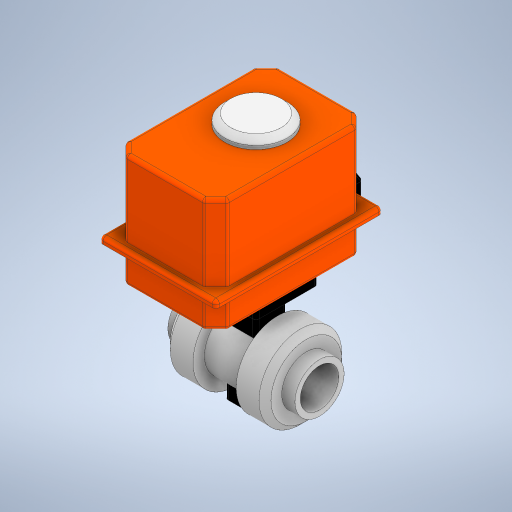
# Autodesk Inventor part: СДР 080 Электроклапан
Saved by Autodesk Inventor 2024.2 (Build 282272000, 272)
## iProperties
Created: 2024-04-05
Part Number: СДР 080 Электроклапан
Material: Generic
Document SubType Name: Modeling
Designer: pokla
Density: 1 g/cm^3
Appearance: Default
Author: pokla
Autodesk Inventor part; units mm, degrees
ref_plane "YZ Plane" through (0, 0, 0) normal (1, 0, 0) x (0, 1, 0)
ref_plane "XZ Plane" through (0, 0, 0) normal (0, 1, 0) x (-1, 0, 0)
ref_plane "XY Plane" through (0, 0, 0) normal (0, 0, 1) x (1, 0, 0)
sketch "Sketch1" plane through (0, 0, 0) normal (0, 1, 0) x (-1, 0, 0)
  line L0 (1079.5, -1295.4) -> (-1079.5, -1295.4)
  line L1 (-1079.5, -1295.4) -> (-1079.5, 1930.4)
  line L2 (-1079.5, 1930.4) -> (1079.5, 1930.4)
  line L3 (1079.5, 1930.4) -> (1079.5, -1295.4)
  line L4 (-1231.9, -1447.8) -> (1231.9, -1447.8)
  line L5 (1231.9, -1447.8) -> (1231.9, 2082.8)
  line L6 (1231.9, 2082.8) -> (-1231.9, 2082.8)
  line L7 (-1231.9, 2082.8) -> (-1231.9, -1447.8)
  point P0 (0, 0)
  point P1 (0, -1295.4)
  dimension "d0" = 2159
  dimension "d1" = 3225.8
  dimension "d5" = 1295.4
  dimension "d6" = 152.4
  constraints: 16 end point, 4 parallel, 2 perpendicular, 1 horizontal, 1 midpoint, 1 vertical alignment, 3 other
  measures "d0" distance of L1.end L2.end
  measures "d1" distance of L0.end L1.end
  measures "d5" distance of point (0, 0) point (0, -1295.4)
  measures "d6" distance between parallel lines of L0 L4
extrude "Extrusion1" add sketch "Sketch1" along normal mid plane 139.7 contours L0 L1 L2 L3 | L7 L6 L5 L4
sketch "Sketch2" plane through (0, 0, 0) normal (0, 1, 0) x (-1, 0, 0)
  line L0 (1231.9, -1447.8) -> (1231.9, 2082.8) projected
  line L1 (1231.9, 2082.8) -> (-1231.9, 2082.8) projected
  line L2 (-1231.9, 2082.8) -> (-1231.9, -1447.8) projected
  line L3 (-1231.9, -1447.8) -> (1231.9, -1447.8) projected
  line L4 (1079.5, -1295.4) -> (1079.5, 1930.4)
  line L5 (1079.5, 1930.4) -> (-1079.5, 1930.4)
  line L6 (-1079.5, 1930.4) -> (-1079.5, -1295.4)
  line L7 (-1079.5, -1295.4) -> (1079.5, -1295.4)
  point P0 (0, 0)
  dimension "d9" = 152.4
  constraints: 8 end point, 3 other
  measures "d9" distance between parallel lines of L3 L7
extrude "Extrusion2" add sketch "Sketch2" along normal blind 1676.4 and the other way blind 736.6 contours L7 L6 L5 L4
sketch "Sketch3" plane through (0, 0, 0) normal (0, 1, 0) x (-1, 0, 0)
  circle A0 centre (0, 0) radius 660.4
  line L0 (1231.9, -1447.8) -> (-1231.9, -1447.8) projected
  line L1 (1079.5, 1930.4) -> (-1079.5, 1930.4) projected
  line L2 (-1079.5, 1930.4) -> (-1079.5, -1295.4) projected
  line L3 (-1079.5, -1295.4) -> (1079.5, -1295.4) projected
  line L4 (1079.5, -1295.4) -> (1079.5, 1930.4) projected
  point P0 (0, 0)
  point P1 (0, -1447.8)
  point P2 (0, -1295.4)
  dimension "d14" = 1320.8
  dimension "d16" = 1295.4
  constraints: 2 midpoint, 1 centre point, 1 coincident
  measures "d14" diameter of A0
  measures "d16" distance of A0.centre point (0, -1295.4)
extrude "Extrusion3" add sketch "Sketch3" along normal blind 1879.6 and the other way blind 12.7 contours A0
sketch "Sketch4" plane through (0, 0, 0) normal (0, 1, 0) x (-1, 0, 0)
  line L0 (685.8, -685.8) -> (-685.8, -685.8)
  line L1 (-685.8, -685.8) -> (-685.8, 685.8)
  line L2 (-685.8, 685.8) -> (685.8, 685.8)
  line L3 (685.8, 685.8) -> (685.8, -685.8)
  circle A0 centre (0, 0) radius 660.4 projected
  line L4 (1079.5, 1930.4) -> (-1079.5, 1930.4) projected
  line L5 (-1079.5, 1930.4) -> (-1079.5, -1295.4) projected
  line L6 (-1079.5, -1295.4) -> (1079.5, -1295.4) projected
  line L7 (1079.5, -1295.4) -> (1079.5, 1930.4) projected
  point P0 (0, 0)
  point P1 (0, -685.8)
  point P2 (0, -1295.4)
  dimension "d21" = 1371.6
  dimension "d22" = 1371.6
  dimension "d23" = 609.6
  constraints: 8 end point, 2 midpoint, 2 parallel, 1 horizontal, 1 perpendicular, 1 vertical alignment
  measures "d21" distance of L1.end L2.end
  measures "d22" distance of L0.end L1.end
  measures "d23" distance of point (0, -685.8) point (0, -1295.4)
extrude "Extrusion4" add sketch "Sketch4" against normal blind 990.6 contours L0 L1 L2 L3 | A0
sketch "Sketch5" plane through (0, 0, 0) normal (0, 1, 0) x (-1, 0, 0)
  line L0 (-685.8, 685.8) -> (685.8, 685.8) projected
  line L1 (685.8, 685.8) -> (685.8, -685.8) projected
  line L2 (685.8, -685.8) -> (-685.8, -685.8) projected
  line L3 (-685.8, -685.8) -> (-685.8, 685.8) projected
  line L4 (-660.4, -660.4) -> (660.4, -660.4)
  line L5 (660.4, -660.4) -> (660.4, 660.4)
  line L6 (660.4, 660.4) -> (-660.4, 660.4)
  line L7 (-660.4, 660.4) -> (-660.4, -660.4)
  point P0 (0, 0)
  dimension "d26" = 25.4
  constraints: 8 end point, 3 other
  measures "d26" distance between parallel lines of L2 L4
extrude "Extrusion5" add sketch "Sketch5" against normal blind 1270 contours L7 L6 L5 L4
sketch "Sketch6" plane through (0, 0, 0) normal (0, 1, 0) x (-1, 0, 0)
  line L0 (660.4, 660.4) -> (660.4, -660.4) projected
  line L1 (660.4, -660.4) -> (-660.4, -660.4) projected
  line L2 (-660.4, -660.4) -> (-660.4, 660.4) projected
  line L3 (-660.4, 660.4) -> (660.4, 660.4) projected
  line L4 (-330.2, -330.2) -> (330.2, -330.2)
  line L5 (330.2, -330.2) -> (330.2, 330.2)
  line L6 (330.2, 330.2) -> (-330.2, 330.2)
  line L7 (-330.2, 330.2) -> (-330.2, -330.2)
  point P0 (0, 0)
  dimension "d29" = 330.2
  constraints: 8 end point, 3 other
  measures "d29" distance between parallel lines of L1 L4
extrude "Extrusion6" add sketch "Sketch6" against normal blind 3352.8 contours L7 L6 L5 L4
sketch "Sketch7" plane through (0, 0, 0) normal (1, 0, 0) x (0, 1, 0)
  line L0 (-1270, -330.2) -> (-1270, 330.2) projected
  line L1 (-1270, -330.2) -> (-3352.8, -330.2) projected
  line L2 (-3352.8, 330.2) -> (-3352.8, -330.2) projected
  line L3 (-1270, 330.2) -> (-3352.8, 330.2) projected
  circle A0 centre (-2489.2, 0) radius 635
  point P0 (0, 0)
  point P1 (-1270, 0)
  dimension "d32" = 1270
  dimension "d33" = 1219.2
  constraints: 1 centre point, 1 horizontal alignment, 1 midpoint
  measures "d32" diameter of A0
  measures "d33" distance of point (-1270, 0) A0.centre
extrude "Extrusion7" add sketch "Sketch7" along normal mid plane 914.4 contours A0 L1 | L1 A0 L3 | L3 A0
sketch "Sketch8" plane through (0, 0, 0) normal (1, 0, 0) x (0, 1, 0)
  circle A0 centre (-2489.2, 0) radius 635 projected
  circle A1 centre (-2489.2, 0) radius 406.4
  circle A2 centre (-2489.2, 0) radius 520.7
  point P0 (0, 0)
  dimension "d36" = 812.8
  dimension "d37" = 1041.4
  constraints: 2 centre point, 2 coincident
  measures "d36" diameter of A1
  measures "d37" diameter of A2
extrude "Extrusion8" add sketch "Sketch8" along normal mid plane 2692.4 contours A2
sketch "Sketch9" plane through (-457.2, -2489.2, 0) normal (-1, 0, 0) x (0, 0, 1)
  circle A0 centre (0, 0) radius 406.4 projected
  circle A1 centre (0, 0) radius 876.3
  point P0 (0, 2489.2)
  dimension "d40" = 1752.6
  constraints: 1 centre point, 1 coincident
  measures "d40" diameter of A1
extrude "Extrusion9" add sketch "Sketch9" along normal blind 609.6
chamfer "Chamfer1" distance 127 angle 45 1 edges at (-1066.8, -2489.2, -876.3)
mirror "Mirror1" about plane through (0, 0, 0) normal (1, 0, 0) of "Extrusion9", "Chamfer1"
sketch "Sketch10" plane through (0, 0, 0) normal (0, 0, 1) x (1, 0, 0)
  line L0 (-1231.9, -69.85) -> (1231.9, -69.85) projected
  line L1 (1079.5, -69.85) -> (-1079.5, -69.85) projected
  line L2 (1079.5, -736.6) -> (1079.5, -69.85) projected
  line L3 (-1079.5, -736.6) -> (1079.5, -736.6) projected
  line L4 (-1079.5, -736.6) -> (-1079.5, -69.85) projected
  line L5 (304.8, -69.85) -> (304.8, -374.65)
  arc A0 (-304.8, -374.65) -> (304.8, -374.65) centre (0, -374.65) ccw
  line L6 (-304.8, -374.65) -> (-304.8, -69.85)
  point P0 (0, 0)
  point P1 (0, -679.45)
  point P2 (0, -69.85)
  point P3 (-304.8, -69.85)
  dimension "d46" = 609.6
  dimension "d47" = 609.6
  constraints: 4 end point, 3 point on circle, 2 perpendicular, 2 point on line, 2 tangent, 1 centre point, 1 midpoint, 1 vertical alignment
  measures "d46" distance between parallel lines of L6 L5
  measures "d47" distance of point (0, -69.85) point (0, -679.45)
extrude "Extrusion10" add sketch "Sketch10" against normal blind 1422.4 contours L0 L5 A0 L6
sketch "Sketch11" plane through (0, 0, 0) normal (0, 0, 1) x (1, 0, 0)
  line L0 (304.8, -69.85) -> (304.8, -374.65) projected
  arc A0 (-304.8, -374.65) -> (304.8, -374.65) centre (0, -374.65) ccw projected
  line L1 (-304.8, -374.65) -> (-304.8, -69.85) projected
  line L2 (304.8, -69.85) -> (-304.8, -69.85) projected
  line L3 (0, -66.6914) -> (266.7, -220.6707)
  line L4 (266.7, -220.6707) -> (266.7, -528.6293)
  line L5 (266.7, -528.6293) -> (0, -682.6086)
  line L6 (0, -682.6086) -> (-266.7, -528.6293)
  line L7 (-266.7, -528.6293) -> (-266.7, -220.6707)
  line L8 (-266.7, -220.6707) -> (0, -66.6914)
  point P0 (0, 0)
  dimension "d50" = 533.4
  constraints: 12 end point, 1 coincident, 1 parallel, 13 other
  measures "d50" distance between parallel lines of L7 L4
extrude "Extrusion11" add sketch "Sketch11" against normal blind 2082.8 contours L3 L4 A0 L5 L6 L7 L8 L2 | L2 L8 L3 | L4 L5 A0 | L5 L6 A0 | A0 L6 L7
chamfer "Chamfer2" distance 127 angle 45 6 edges at (-133.35, -143.681, -2082.8) (133.35, -143.681, -2082.8) (266.7, -374.65, -2082.8) (133.35, -605.619, -2082.8) (-133.35, -605.619, -2082.8) (-266.7, -374.65, -2082.8)
chamfer "Chamfer3" distance 127 angle 45 1 edges at (660.4, 1879.6, 0)
sketch "Sketch12" plane through (0, 0, 0) normal (0, 1, 0) x (-1, 0, 0)
  line L0 (-685.8, 685.8) -> (-685.8, -685.8) projected
  line L1 (-685.8, -685.8) -> (685.8, -685.8) projected
  line L2 (685.8, -685.8) -> (685.8, 685.8) projected
  line L3 (685.8, 685.8) -> (-685.8, 685.8) projected
  line L4 (-1079.5, 1930.4) -> (1079.5, 1930.4) projected
  line L5 (1079.5, 1930.4) -> (1079.5, -1295.4) projected
  line L6 (1079.5, -1295.4) -> (-1079.5, -1295.4) projected
  line L7 (-1079.5, -1295.4) -> (-1079.5, 1930.4) projected
  circle A0 centre (165.1, 1092.2) radius 101.6
  circle A1 centre (165.1, 1092.2) radius 63.5
  point P0 (0, 0)
  dimension "d59" = 203.2
  dimension "d60" = 914.4
  dimension "d61" = 838.2
  dimension "d62" = 127
  constraints: 2 centre point, 1 coincident
  measures "d59" diameter of A0
  measures "d60" distance from line of L5 A0.centre
  measures "d61" distance from line of L4 A0.centre
  measures "d62" diameter of A1
extrude "Extrusion12" add sketch "Sketch12" against normal blind 990.6 contours A0
chamfer "Chamfer4" distance 254 angle 45 8 edges at (1079.5, 873.125, 1930.4) (1079.5, 873.125, -1295.4) (1079.5, -403.225, -1295.4) (1079.5, -403.225, 1930.4) (-1079.5, -403.225, -1295.4) (-1079.5, 873.125, -1295.4) (-1079.5, -403.225, 1930.4) (-1079.5, 873.125, 1930.4)
fillet "Fillet1" radius 76.2 32 edges at (-1079.5, 1676.4, 317.5) (0, 1676.4, -1295.4) (0, 1676.4, 1930.4) (1079.5, 1676.4, 317.5) (-952.5, 1676.4, 1803.4) (952.5, 1676.4, 1803.4) (952.5, 1676.4, -1168.4) (-952.5, 1676.4, -1168.4) (-952.5, -736.6, 1803.4) (0, -736.6, 1930.4) (952.5, -736.6, 1803.4) (1079.5, -736.6, 317.5) (952.5, -736.6, -1168.4) (0, -736.6, -1295.4) (-952.5, -736.6, -1168.4) (-1079.5, -736.6, 317.5) (825.5, 873.125, -1295.4) (1079.5, 873.125, -1041.4) (825.5, -403.225, -1295.4) (1079.5, -403.225, -1041.4) (-825.5, 873.125, -1295.4) (-1079.5, 873.125, -1041.4) (-1079.5, -403.225, -1041.4) (-825.5, -403.225, -1295.4) (-825.5, 873.125, 1930.4) (-1079.5, 873.125, 1676.4) (-825.5, -403.225, 1930.4) (-1079.5, -403.225, 1676.4) (1079.5, 873.125, 1676.4) (825.5, 873.125, 1930.4) (1079.5, -403.225, 1676.4) (825.5, -403.225, 1930.4)
fillet "Fillet2" radius 76.2 8 edges at (-1231.9, 0, -1447.8) (0, 69.85, -1447.8) (-1231.9, 69.85, 317.5) (1231.9, 0, -1447.8) (1231.9, 69.85, 317.5) (1231.9, 0, 2082.8) (0, 69.85, 2082.8) (-1231.9, 0, 2082.8)
fillet "Fillet3" radius 76.2 16 edges at (685.8, -863.6, -685.8) (660.4, -1130.3, -660.4) (-685.8, -863.6, -685.8) (-660.4, -1130.3, -660.4) (-685.8, -863.6, 685.8) (-660.4, -1130.3, 660.4) (685.8, -863.6, 685.8) (660.4, -1130.3, 660.4) (330.2, -1608.4022, 330.2) (330.2, -1608.4022, -330.2) (-330.2, -1608.4022, -330.2) (-330.2, -1608.4022, 330.2) (-330.2, -3192.1978, 330.2) (330.2, -3192.1978, 330.2) (330.2, -3192.1978, -330.2) (-330.2, -3192.1978, -330.2)
body "Solid1"
